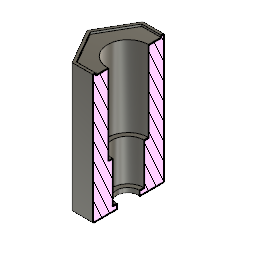
ConnectorStandJig (Autodesk Fusion 360 design; units mm, degrees)
Autodesk Fusion 360 part; units mm, degrees
sketch "Sketch1" plane through (0, 0, 0) normal (0, 0, 1) x (1, 0, 0)
  line L0 (-9.0933, 15.75) -> (-18.1865, 0)
  line L1 (-18.1865, 0) -> (-9.0933, -15.75)
  line L2 (-9.0933, -15.75) -> (9.0933, -15.75)
  line L3 (9.0933, -15.75) -> (18.1865, 0)
  line L4 (18.1865, 0) -> (9.0933, 15.75)
  line L5 (9.0933, 15.75) -> (-9.0933, 15.75)
  dimension "d8" = 31.5
  measures "d8" distance of L2 L5
extrude "Extrude1" add sketch "Sketch1" along normal blind 56.1
sketch "Sketch3" plane through (0, 0, 56.1) normal (0, 0, 1) x (-1, 0, 0)
  line L0 (-9.0933, -15.75) -> (9.0933, -15.75)
  line L1 (9.0933, -15.75) -> (18.1865, 0)
  line L2 (18.1865, 0) -> (9.0933, 15.75)
  line L3 (9.0933, 15.75) -> (-9.0933, 15.75)
  line L4 (-9.0933, 15.75) -> (-18.1865, 0)
  line L5 (-18.1865, 0) -> (-9.0933, -15.75)
hole "Hole1" at (0, 0, 56.1) direction (0, 0, -1) diameter 18 end through all
sketch "Sketch4" plane through (0, 0, 0) normal (0, 0, -1) x (1, 0, 0)
  circle A0 centre (0, 0) radius 9
  line L0 (-9.0933, -15.75) -> (9.0933, -15.75)
  line L1 (9.0933, -15.75) -> (18.1865, 0)
  line L2 (18.1865, 0) -> (9.0933, 15.75)
  line L3 (9.0933, 15.75) -> (-9.0933, 15.75)
  line L4 (-9.0933, 15.75) -> (-18.1865, 0)
  line L5 (-18.1865, 0) -> (-9.0933, -15.75)
  circle A1 centre (0, 0) radius 9
  circle A2 centre (0, 0) radius 5
  dimension "d12" = 10
  constraint concentric A1 A2
  measures "d12" diameter of A2
extrude "Extrude3" add sketch "Sketch4" against normal blind 2.1 contours A0 A1
sketch "Sketch5" plane through (0, 0, 56.1) normal (0, 0, 1) x (-1, 0, 0)
  circle A0 centre (0, 0) radius 9
  line L0 (-9.0933, -15.75) -> (9.0933, -15.75)
  line L1 (9.0933, -15.75) -> (18.1865, 0)
  line L2 (18.1865, 0) -> (9.0933, 15.75)
  line L3 (9.0933, 15.75) -> (-9.0933, 15.75)
  line L4 (-9.0933, 15.75) -> (-18.1865, 0)
  line L5 (-18.1865, 0) -> (-9.0933, -15.75)
  line L6 (8.4004, -14.55) -> (16.8009, 0)
  line L7 (16.8009, 0) -> (8.4004, 14.55)
  line L8 (8.4004, 14.55) -> (-8.4004, 14.55)
  line L9 (-8.4004, 14.55) -> (-16.8009, 0)
  line L10 (-16.8009, 0) -> (-8.4004, -14.55)
  line L11 (-8.4004, -14.55) -> (8.4004, -14.55)
  dimension "d15" = 29.1
  constraint coincident A0.centre origin
  measures "d15" distance of L8 L11
extrude "Extrude4" add sketch "Sketch5" along normal blind 0.9 contours L0 L1 L2 L3 L4 L5
sketch "Sketch6" plane through (0, 0, 0) normal (0, 0, -1) x (-1, 0, 0)
  line L0 (8.4004, -14.55) -> (-8.4004, -14.55)
  line L1 (-8.4004, -14.55) -> (-16.8009, 0)
  line L2 (-16.8009, 0) -> (-8.4004, 14.55)
  line L3 (-8.4004, 14.55) -> (8.4004, 14.55)
  line L4 (8.4004, 14.55) -> (16.8009, 0)
  line L5 (16.8009, 0) -> (8.4004, -14.55)
  line L6 (-18.1865, 0) -> (-9.0933, -15.75)
  line L7 (-9.0933, -15.75) -> (9.0933, -15.75)
  line L8 (9.0933, -15.75) -> (18.1865, 0)
  line L9 (18.1865, 0) -> (9.0933, 15.75)
  line L10 (9.0933, 15.75) -> (-9.0933, 15.75)
  line L11 (-9.0933, 15.75) -> (-18.1865, 0)
  circle A0 centre (0, 0) radius 7
  circle A1 centre (0, 0) radius 9
  circle A2 centre (0, 0) radius 5
  line L12 (9.0933, 15.75) -> (-9.0933, 15.75)
  line L13 (-9.0933, 15.75) -> (-18.1865, 0)
  line L14 (-18.1865, 0) -> (-9.0933, -15.75)
  line L15 (-9.0933, -15.75) -> (9.0933, -15.75)
  line L16 (9.0933, -15.75) -> (18.1865, 0)
  line L17 (18.1865, 0) -> (9.0933, 15.75)
  dimension "d18" = 14
  constraint coincident A0.centre A1.centre
  measures "d18" diameter of A0
extrude "Extrude5" add sketch "Sketch6" against normal blind 20.4 contours A1
equation "d8 = 29.1 mm + 2.4 mm"
